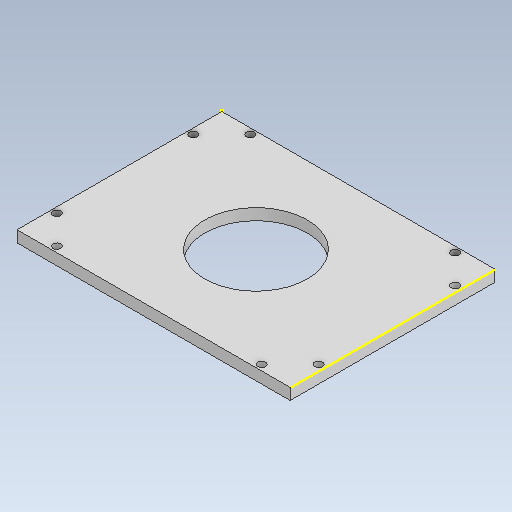
# Autodesk Inventor part: expo2
Saved by Autodesk Inventor 2020 (Build 240168000, 168)
## iProperties
Created: 2020-02-17
Part Number: expo2
Material: Generic
Document SubType Name: Modeling
Designer: Aryan
Density: 1 g/cm^3
Appearance: Default
Author: Aryan
Autodesk Inventor part; units mm, degrees
ref_plane "YZ Plane" through (0, 0, 0) normal (1, 0, 0) x (0, 1, 0)
ref_plane "XZ Plane" through (0, 0, 0) normal (0, 1, 0) x (-1, 0, 0)
ref_plane "XY Plane" through (0, 0, 0) normal (0, 0, 1) x (1, 0, 0)
sketch "Sketch1" plane through (0, 0, 0) normal (0, 1, 0) x (-1, 0, 0)
  line L0 (0, 0) -> (-120, 0)
  line L1 (-120, 0) -> (-120, 90)
  line L2 (-120, 90) -> (0, 90)
  line L3 (0, 90) -> (0, 0)
  line L4 (0, 0) -> (-60, 0)
  line L5 (-60, 0) -> (-60, 45)
  line L6 (-60, 45) -> (0, 45)
  line L7 (0, 45) -> (0, 0)
  circle A0 centre (-60, 45) radius 22.5
  dimension "d0" = 120
  dimension "d1" = 90
  dimension "d2" = 60
  dimension "d3" = 45
  dimension "d4" = 45
  constraints: 16 end point, 4 parallel, 2 horizontal, 2 perpendicular, 1 centre point, 1 coincident
  measures "d0" distance of L1.end L2.end
  measures "d1" distance of L0.end L1.end
  measures "d2" distance of L5.end L6.end
  measures "d3" distance of L4.end L5.end
  measures "d4" diameter of A0
extrude "Extrusion1" add sketch "Sketch1" against normal blind 5
sketch "Sketch2" plane through (0, 0, 0) normal (0, 1, 0) x (1, 0, 0)
  line L0 (0, -90) -> (0, 0) projected
  line L1 (0, 0) -> (60, 0)
  line L2 (60, 0) -> (60, -45)
  line L3 (60, -45) -> (0, -45)
  line L4 (0, -45) -> (0, 0)
  circle A0 centre (60, -45) radius 22.5
  dimension "d7" = 60
  dimension "d8" = 45
  dimension "d9" = 45
  constraints: 8 end point, 2 parallel, 1 centre point, 1 coincident, 1 horizontal, 1 perpendicular
  measures "d7" distance of L2.end L3.end
  measures "d8" distance of L1.end L2.end
  measures "d9" diameter of A0
extrude "Extrusion2" cut sketch "Sketch2" against normal blind 5 contours A0 L2 L3 | L3 L2 A0
sketch "Sketch3" plane through (0, 0, 0) normal (0, 1, 0) x (1, 0, 0)
  line L0 (0, 0) -> (120, 0) projected
  line L1 (0, 0) -> (15, 0)
  line L2 (15, 0) -> (15, -2.5)
  line L3 (15, -2.5) -> (0, -2.5)
  line L4 (0, -2.5) -> (0, 0)
  circle A0 centre (15, -2.5) radius 1.75
  dimension "d12" = 15
  dimension "d13" = 2.5
  dimension "d14" = 3.5
  constraints: 8 end point, 2 parallel, 1 centre point, 1 coincident, 1 horizontal, 1 perpendicular
  measures "d12" distance of L2.end L3.end
  measures "d13" distance of L1.end L2.end
  measures "d14" diameter of A0
extrude "Extrusion3" cut sketch "Sketch3" against normal blind 5 contours A0 L3 L2 | L2 L3 A0
sketch "Sketch4" plane through (0, 0, 0) normal (0, 1, 0) x (1, 0, 0)
  line L0 (120, -90) -> (0, -90) projected
  line L1 (0, -90) -> (15, -90)
  line L2 (15, -90) -> (15, -87.5)
  line L3 (15, -87.5) -> (0, -87.5)
  line L4 (0, -87.5) -> (0, -90)
  circle A0 centre (15, -87.5) radius 1.75
  point P0 (0, 0)
  dimension "d17" = 15
  dimension "d18" = 2.5
  dimension "d19" = 3.5
  constraints: 8 end point, 2 parallel, 1 centre point, 1 coincident, 1 horizontal, 1 perpendicular
  measures "d17" distance of L3.end L2.end
  measures "d18" distance of L2.end L1.end
  measures "d19" diameter of A0
extrude "Extrusion4" cut sketch "Sketch4" against normal blind 5 contours A0 L3 L2 | L2 L3 A0
sketch "Sketch5" plane through (0, 0, 0) normal (0, 1, 0) x (1, 0, 0)
  line L0 (120, 0) -> (120, -90) projected
  line L1 (120, 0) -> (105, 0)
  line L2 (105, 0) -> (105, -2.5)
  line L3 (105, -2.5) -> (120, -2.5)
  line L4 (120, -2.5) -> (120, 0)
  circle A0 centre (105, -2.5) radius 1.75
  point P0 (0, 0)
  dimension "d22" = 15
  dimension "d23" = 2.5
  dimension "d32" = 3.5
  constraints: 8 end point, 2 parallel, 1 centre point, 1 coincident, 1 horizontal, 1 perpendicular
  measures "d22" distance of L3.end L2.end
  measures "d23" distance of L2.end L1.end
  measures "d32" diameter of A0
extrude "Extrusion5" [suppressed]
sketch "Sketch6" plane through (0, 0, 0) normal (0, 1, 0) x (1, 0, 0)
  line L0 (120, 0) -> (120, -90) projected
  line L1 (120, -90) -> (105, -90)
  line L2 (105, -90) -> (105, -87.5)
  line L3 (105, -87.5) -> (120, -87.5)
  line L4 (120, -87.5) -> (120, -90)
  circle A0 centre (105, -87.5) radius 1.75
  point P0 (0, 0)
  dimension "d27" = 15
  dimension "d28" = 2.5
  dimension "d29" = 3.5
  constraints: 8 end point, 2 parallel, 1 centre point, 1 coincident, 1 horizontal, 1 perpendicular
  measures "d27" distance of L2.end L3.end
  measures "d28" distance of L1.end L2.end
  measures "d29" diameter of A0
extrude "Extrusion6" cut sketch "Sketch6" against normal blind 5 contours A0 L2 L3 | L3 L2 A0
sketch "Sketch7" plane through (0, 0, 0) normal (0, 1, 0) x (1, 0, 0)
  line L0 (0, 0) -> (120, 0) projected
  line L1 (120, 0) -> (105, 0)
  line L2 (105, 0) -> (105, -2.5)
  line L3 (105, -2.5) -> (120, -2.5)
  line L4 (120, -2.5) -> (120, 0)
  circle A0 centre (105, -2.5) radius 1.75
  dimension "d33" = 15
  dimension "d34" = 2.5
  dimension "d35" = 3.5
  constraints: 8 end point, 2 parallel, 1 centre point, 1 coincident, 1 horizontal, 1 perpendicular
  measures "d33" distance of L3.end L2.end
  measures "d34" distance of L2.end L1.end
  measures "d35" diameter of A0
extrude "Extrusion7" cut sketch "Sketch7" against normal blind 5 contours A0 L3 L2 | L2 L3 A0
sketch "Sketch8" plane through (0, 0, 0) normal (0, 1, 0) x (1, 0, 0)
  line L0 (0, 0) -> (2.5, 0)
  line L1 (2.5, 0) -> (2.5, -15)
  line L2 (2.5, -15) -> (0, -15)
  line L3 (0, -15) -> (0, 0)
  circle A0 centre (2.5, -15) radius 1.75
  dimension "d38" = 2.5
  dimension "d39" = 15
  dimension "d40" = 3.5
  constraints: 8 end point, 2 parallel, 1 centre point, 1 coincident, 1 horizontal, 1 perpendicular
  measures "d38" distance of L1.end L2.end
  measures "d39" distance of L0.end L1.end
  measures "d40" diameter of A0
extrude "Extrusion8" cut sketch "Sketch8" against normal blind 10 contours A0 L2 L1 | L1 L2 A0
sketch "Sketch9" plane through (0, 0, 0) normal (0, 1, 0) x (1, 0, 0)
  line L0 (0, -90) -> (2.5, -90)
  line L1 (2.5, -90) -> (2.5, -75)
  line L2 (2.5, -75) -> (0, -75)
  line L3 (0, -75) -> (0, -90)
  circle A0 centre (2.5, -75) radius 1.75
  point P0 (0, 0)
  dimension "d43" = 2.5
  dimension "d44" = 15
  dimension "d45" = 3.5
  constraints: 8 end point, 2 parallel, 1 centre point, 1 coincident, 1 horizontal, 1 perpendicular
  measures "d43" distance of L2.end L1.end
  measures "d44" distance of L1.end L0.end
  measures "d45" diameter of A0
extrude "Extrusion9" cut sketch "Sketch9" against normal blind 10 contours A0 L2 L1 | L1 L2 A0
sketch "Sketch10" plane through (0, 0, 0) normal (0, 1, 0) x (1, 0, 0)
  line L0 (120, 0) -> (120, -90) projected
  point P0 (0, 0)
sketch "Sketch11" plane through (0, 0, 0) normal (0, 1, 0) x (1, 0, 0)
  line L0 (120, 0) -> (120, -90) projected
  line L1 (120, 0) -> (117.5, 0)
  line L2 (117.5, 0) -> (117.5, -15)
  line L3 (117.5, -15) -> (120, -15)
  line L4 (120, -15) -> (120, 0)
  circle A0 centre (117.5, -15) radius 1.75
  point P0 (0, 0)
  dimension "d50" = 2.5
  dimension "d51" = 15
  dimension "d52" = 3.5
  constraints: 8 end point, 2 parallel, 1 centre point, 1 coincident, 1 horizontal, 1 perpendicular
  measures "d50" distance of L3.end L2.end
  measures "d51" distance of L2.end L1.end
  measures "d52" diameter of A0
extrude "Extrusion10" cut sketch "Sketch11" against normal blind 10 contours A0 L2 L3 | L3 L2 A0
sketch "Sketch12" plane through (0, 0, 0) normal (0, 1, 0) x (1, 0, 0)
  line L0 (120, -90) -> (0, -90) projected
  line L1 (120, -90) -> (117.5, -90)
  line L2 (117.5, -90) -> (117.5, -75)
  line L3 (117.5, -75) -> (120, -75)
  line L4 (120, -75) -> (120, -90)
  circle A0 centre (117.5, -75) radius 1.75
  point P0 (0, 0)
  dimension "d55" = 2.5
  dimension "d56" = 15
  dimension "d57" = 3.5
  constraints: 8 end point, 2 parallel, 1 centre point, 1 coincident, 1 horizontal, 1 perpendicular
  measures "d55" distance of L2.end L3.end
  measures "d56" distance of L1.end L2.end
  measures "d57" diameter of A0
extrude "Extrusion11" cut sketch "Sketch12" against normal blind 10 contours A0 L3 L2 | L2 L3 A0
body "Solid1"
